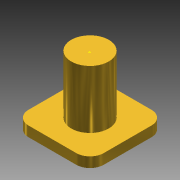
# Autodesk Inventor part: BNC_Up
Saved by Autodesk Inventor 2014 (Build 180170000, 170)
## iProperties
Created: 2015-01-07
Part Number: BNC_Up
Material: Generic
Document SubType Name: Modeling
Designer: Owner
Density: 1 g/cm^3
Appearance: Gold - Metal
Author: Owner
Autodesk Inventor part; units mm, degrees
ref_plane "YZ Plane" through (0, 0, 0) normal (1, 0, 0) x (0, 1, 0)
ref_plane "XZ Plane" through (0, 0, 0) normal (0, 1, 0) x (-1, 0, 0)
ref_plane "XY Plane" through (0, 0, 0) normal (0, 0, 1) x (1, 0, 0)
sketch "Sketch1" plane through (0, 0, 0) normal (0, 1, 0) x (-1, 0, 0)
  line L0 (-6.3389, 5.775) -> (11.1611, 5.775)
  line L1 (11.1611, 5.775) -> (11.1611, -11.725)
  line L2 (11.1611, -11.725) -> (-6.3389, -11.725)
  line L3 (-6.3389, -11.725) -> (-6.3389, 5.775)
  point P0 (0, 0)
  dimension "d0" = 17.5
  dimension "d1" = 17.5
  constraints: 8 end point, 2 parallel, 1 horizontal, 1 perpendicular
  measures "d0" distance of L0.start L0.end
  measures "d1" distance of L0.end L1.end
extrude "Extrusion1" add sketch "Sketch1" along normal blind 2.36
sketch "Sketch2" plane through (0, 2.36, 0) normal (0, 1, 0) x (1, 0, 0)
  circle A0 centre (-2.4111, 2.975) radius 4.3815
  point P0 (0, 0)
  dimension "d4" = 8.763
  constraints: 1 centre point
  measures "d4" diameter of A0
extrude "Extrusion2" add sketch "Sketch2" along normal blind 13.52
fillet "Fillet1" radius 3.175 4 edges at (6.3389, 1.18, 5.775) (-11.1611, 1.18, 5.775) (6.3389, 1.18, -11.725) (-11.1611, 1.18, -11.725)
body "Solid1"
